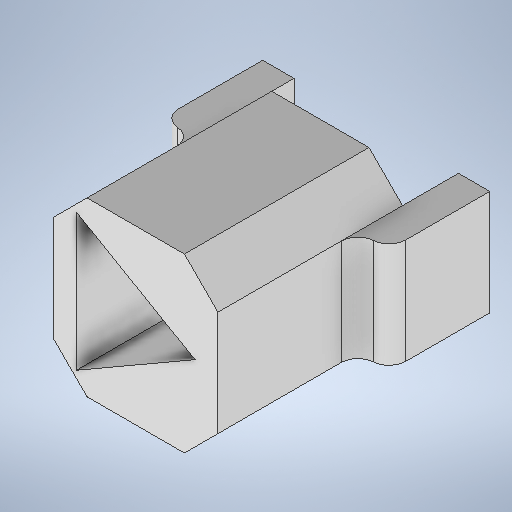
# Autodesk Inventor part: CameraSupportTemp
Saved by Autodesk Inventor 2025.1 (Build 291241000, 241)
## iProperties
Created: 2025-04-03
Part Number: CameraSupportTemp
Material: Generic
Document SubType Name: Modeling
Designer: victo
Density: 1 g/cm^3
Appearance: Default
Author: victo
Autodesk Inventor part; units mm, degrees
ref_plane "YZ Plane" through (0, 0, 0) normal (1, 0, 0) x (0, 1, 0)
ref_plane "XZ Plane" through (0, 0, 0) normal (0, 1, 0) x (-1, 0, 0)
ref_plane "XY Plane" through (0, 0, 0) normal (0, 0, 1) x (1, 0, 0)
sketch "Sketch1" plane through (0, 0, 0) normal (0, 0, 1) x (1, 0, 0)
  line L0 (-20.3, 9.4) -> (20.3, 9.4)
  line L1 (20.3, 9.4) -> (20.3, -9.4)
  line L2 (20.3, -9.4) -> (-20.3, -9.4)
  line L3 (-20.3, -9.4) -> (-20.3, 9.4)
  line L4 (-14.7, 9.4) -> (14.7, 9.4)
  line L5 (14.7, 9.4) -> (14.7, -9.4)
  line L6 (14.7, -9.4) -> (-14.7, -9.4)
  line L7 (-14.7, -9.4) -> (-14.7, 9.4)
  point P0 (0, 0)
  point P1 (14.7, 9.4)
  dimension "d0" = 29.4
  dimension "d1" = 18.8
  dimension "d2" = 9.4
  dimension "d3" = 14.7
  dimension "d4" = 5.6
  dimension "d5" = 5.6
  constraints: 16 end point, 4 parallel, 2 horizontal, 2 perpendicular, 2 point on line
  measures "d0" distance between parallel lines of L5 L7
  measures "d1" distance between parallel lines of L0 L2
  measures "d2" distance from line of L2 point (0, 0)
  measures "d3" distance from line of point (0, 0) L5
  measures "d4" distance between parallel lines of L7 L3
  measures "d5" distance between parallel lines of L5 L1
extrude "Extrusion1" add sketch "Sketch1" along normal blind 18
extrude "Extrusion2" cut sketch "Sketch1" along normal blind 10 contours L0 L5 L2 L7
sketch "Sketch2" plane through (0, 0, 18) normal (0, 0, 1) x (1, 0, 0)
  line L0 (10.6, 0) -> (-10.6, 12.2398)
  line L1 (-10.6, 12.2398) -> (-10.6, -12.2398)
  line L2 (14.7, 9.4) -> (-14.7, 9.4) projected
  line L3 (-10.6, -12.2398) -> (10.6, 0)
  line L4 (-20.3, 9.4) -> (-20.3, -9.4) projected
  line L5 (14.7, -9.4) -> (14.7, 9.4) projected
  line L6 (-14.7, 9.4) -> (-14.7, -9.4) projected
  line L7 (14.7, -9.4) -> (-14.7, -9.4)
  line L8 (-14.7, -9.4) -> (-14.7, -15.4)
  line L9 (-14.7, -15.4) -> (14.7, -15.4)
  line L10 (14.7, -15.4) -> (14.7, -9.4)
  line L11 (14.7, 9.4) -> (-14.7, 9.4)
  line L12 (-14.7, 9.4) -> (-14.7, 15.4)
  line L13 (-14.7, 15.4) -> (14.7, 15.4)
  line L14 (14.7, 15.4) -> (14.7, 9.4)
  point P0 (0, 0)
  point P1 (-10.6, 0)
  point P2 (0, -6.1199)
  point P3 (0, 6.1199)
  point P4 (-14.7, 9.4)
  point P5 (-14.7, -9.4)
  point P6 (-5.6813, -9.4)
  point P7 (-10.6, -9.4)
  point P8 (-10.6, 9.4)
  point P9 (-5.6813, 9.4)
  dimension "d17" = 21.2
  dimension "d18" = 0
  dimension "d19" = 21.2
  dimension "d20" = 21.2
  dimension "d21" = 10.6
  dimension "d25" = 6
  dimension "d26" = 6
  dimension "d27" = 0
  dimension "d28" = 0
  constraints: 22 end point, 5 parallel, 3 midpoint, 3 perpendicular, 2 horizontal
  measures "d17" distance of point (-10.6, 0) L0.start
  measures "d18" vertical distance of point (0, 0) point (-10.6, 0)
  measures "d19" distance of point (0, -6.12) L0.end
  measures "d20" distance of point (0, 6.12) L1.end
  measures "d21" distance of point (0, 0) point (-10.6, 0)
  measures "d25" distance of L8.end L7.end
  measures "d26" distance of L11.end L12.end
  measures "d27" distance between parallel lines of L6 L8
  measures "d28" distance between parallel lines of L6 L12
extrude "Extrusion3" add sketch "Sketch2" along normal blind 10 and the other way blind 8 contours L0 L2 L5 L7 L3 | L0 L1 L2 L12 L13 L14 | L7 L10 L9 L8 L1 L3 | L1 L7 L6 L2
extrude "Extrusion4" add sketch "Sketch2" against normal blind 8 contours L2 L1 L0 | L3 L1 L7
chamfer "Chamfer1" distance 6 angle 45 4 edges at (-14.7, 15.4, 19) (-14.7, -15.4, 19) (14.7, -15.4, 19) (14.7, 15.4, 19)
fillet "Fillet1" radius 3 4 edges at (14.7, 0, 18) (-14.7, 0, 18) (-20.3, 0, 18) (20.3, 0, 18)
sketch "Sketch4" plane through (0, 0, 28) normal (0, 0, 1) x (1, 0, 0)
  line L0 (8.7, 15.4) -> (14.7, 9.4) projected
  line L1 (8.7, 15.4) -> (-8.7, 15.4) projected
  line L2 (-14.7, 9.4) -> (-8.7, 15.4) projected
  line L3 (-14.7, 9.4) -> (-14.7, -9.4) projected
  line L4 (-8.7, -15.4) -> (-14.7, -9.4) projected
  line L5 (-8.7, -15.4) -> (8.7, -15.4) projected
  line L6 (14.7, -9.4) -> (8.7, -15.4) projected
  line L7 (14.7, -9.4) -> (14.7, 9.4) projected
  line L8 (-10.6, 12.2398) -> (10.6, 0) projected
  line L9 (10.6, 0) -> (-10.6, -12.2398) projected
  line L10 (-10.6, -12.2398) -> (-10.6, 12.2398) projected
  point P0 (0, 0)
extrude "Extrusion5" add sketch "Sketch4" along normal blind 15
equation "\"d2\" = 0.5 * d1"
equation "\"d3\" = 0.5 * d0"
equation "\"d5\" = d4"
body "Solid1"
